Autodesk Fusion 360 part; units mm, degrees
note: some values were not read from the file. Set by a fixed rule: which sketch regions a step uses.
(part 2 of 2)
sketch "Sketch32" plane through (0, 0, 0) normal (0, -1, 0) x (1, 0, 0)
  line L0 (30, 47) -> (60, 47)
  line L1 (60, 47) -> (60, 33)
  line L2 (60, 33) -> (30, 33)
  line L3 (30, 33) -> (30, 47)
  line L4 (52, 23) -> (68, 23)
  line L5 (68, 23) -> (68, 13)
  line L6 (68, 13) -> (52, 13)
  line L7 (52, 13) -> (52, 23)
  circle A0 centre (30, 18) radius 5
  line L8 (3, 20) -> (3, 10)
  line L9 (3, 10) -> (0, 10)
  line L10 (0, 10) -> (0, 0)
  line L11 (0, 0) -> (10, 0)
  line L12 (10, 0) -> (10, 3)
  line L13 (10, 3) -> (20, 3)
  line L14 (20, 3) -> (20, 0)
  line L15 (20, 0) -> (30, 0)
  line L16 (30, 0) -> (30, 3)
  line L17 (30, 3) -> (40, 3)
  line L18 (40, 3) -> (40, 0)
  line L19 (40, 0) -> (50, 0)
  line L20 (50, 0) -> (50, 3)
  line L21 (50, 3) -> (60, 3)
  line L22 (60, 3) -> (60, 0)
  line L23 (60, 0) -> (70, 0)
  line L24 (70, 0) -> (70, 3)
  line L25 (70, 3) -> (80, 3)
  line L26 (80, 3) -> (80, 0)
  line L27 (80, 0) -> (90, 0)
  line L28 (90, 0) -> (90, 10)
  line L29 (90, 10) -> (87, 10)
  line L30 (87, 10) -> (87, 20)
  line L31 (87, 20) -> (90, 20)
  line L32 (90, 20) -> (90, 30)
  line L33 (90, 30) -> (87, 30)
  line L34 (87, 30) -> (87, 40)
  line L35 (87, 40) -> (90, 40)
  line L36 (90, 40) -> (90, 50)
  line L37 (90, 50) -> (87, 50)
  line L38 (87, 50) -> (87, 60)
  line L39 (87, 60) -> (90, 60)
  line L40 (90, 60) -> (90, 70)
  line L41 (90, 70) -> (80, 70)
  line L42 (80, 70) -> (80, 67)
  line L43 (80, 67) -> (70, 67)
  line L44 (70, 67) -> (70, 70)
  line L45 (70, 70) -> (60, 70)
  line L46 (60, 70) -> (60, 67)
  line L47 (60, 67) -> (50, 67)
  line L48 (50, 67) -> (50, 70)
  line L49 (50, 70) -> (40, 70)
  line L50 (40, 70) -> (40, 67)
  line L51 (40, 67) -> (30, 67)
  line L52 (30, 67) -> (30, 70)
  line L53 (30, 70) -> (20, 70)
  line L54 (20, 70) -> (20, 67)
  line L55 (20, 67) -> (10, 67)
  line L56 (10, 67) -> (10, 70)
  line L57 (10, 70) -> (0, 70)
  line L58 (0, 70) -> (0, 60)
  line L59 (0, 60) -> (3, 60)
  line L60 (3, 60) -> (3, 50)
  line L61 (3, 50) -> (0, 50)
  line L62 (0, 50) -> (0, 40)
  line L63 (0, 40) -> (3, 40)
  line L64 (3, 40) -> (3, 30)
  line L65 (3, 30) -> (0, 30)
  line L66 (0, 30) -> (0, 20)
  line L67 (0, 20) -> (3, 20)
  circle A1 centre (67, 43) radius 0.5
  circle A2 centre (73, 43) radius 0.5
  circle A3 centre (68.5, 43) radius 0.5
  circle A4 centre (70, 43) radius 0.5
  circle A5 centre (71.5, 43) radius 0.5
  circle A6 centre (67.75, 42) radius 0.5
  circle A7 centre (69.25, 42) radius 0.5
  circle A8 centre (70.75, 42) radius 0.5
  circle A9 centre (72.25, 42) radius 0.5
  circle A10 centre (67, 41) radius 0.5
  circle A11 centre (68.4962, 41) radius 0.5
  circle A12 centre (70, 41) radius 0.5
  circle A13 centre (71.5, 41) radius 0.5
  circle A14 centre (73, 41) radius 0.5
  circle A15 centre (67.75, 40) radius 0.5
  circle A16 centre (69.25, 40) radius 0.5
  circle A17 centre (70.75, 40) radius 0.5
  circle A18 centre (72.25, 40) radius 0.5
  circle A19 centre (67, 39) radius 0.5
  circle A20 centre (68.4962, 39) radius 0.5
  circle A21 centre (70, 39) radius 0.5
  circle A22 centre (71.5, 39) radius 0.5
  circle A23 centre (73, 39) radius 0.5
  circle A24 centre (23, 43) radius 0.5
  circle A25 centre (21.5, 43) radius 0.5
  circle A26 centre (20, 43) radius 0.5
  circle A27 centre (18.5, 43) radius 0.5
  circle A28 centre (17, 43) radius 0.5
  circle A29 centre (17.75, 42) radius 0.5
  circle A30 centre (19.25, 42) radius 0.5
  circle A31 centre (20.75, 42) radius 0.5
  circle A32 centre (22.25, 42) radius 0.5
  circle A33 centre (21.5038, 41) radius 0.5
  circle A34 centre (20, 41) radius 0.5
  circle A35 centre (18.5, 41) radius 0.5
  circle A36 centre (17, 41) radius 0.5
  circle A37 centre (17.75, 40) radius 0.5
  circle A38 centre (20.75, 40) radius 0.5
  circle A39 centre (19.25, 40) radius 0.5
  circle A40 centre (22.25, 40) radius 0.5
  circle A41 centre (23, 41) radius 0.5
  circle A42 centre (23, 39) radius 0.5
  circle A43 centre (21.5038, 39) radius 0.5
  circle A44 centre (20, 39) radius 0.5
  circle A45 centre (18.5, 39) radius 0.5
  circle A46 centre (17, 39) radius 0.5
  point P0 (70, 40)
  dimension "d174" = 1
  dimension "d175" = 1.5
  dimension "d176" = 1.5
  dimension "d177" = 1
  dimension "d178" = 1
  dimension "d179" = 1.5
  dimension "d180" = 1
  dimension "d182" = 2
  dimension "d183" = 1
  dimension "d184" = 1
  dimension "d185" = 1
  dimension "d186" = 1
  dimension "d187" = 1
  dimension "d188" = 2
  dimension "d189" = 1
  dimension "d190" = 1
  dimension "d191" = 1
  dimension "d192" = 1
  dimension "d193" = 2
  dimension "d194" = 1
  dimension "d195" = 1
  dimension "d196" = 1
  dimension "d197" = 1
  dimension "d198" = 1
  measures "d174" diameter of A6
  measures "d175" distance of A6.centre A7.centre
  measures "d176" distance of A7.centre A8.centre
  measures "d177" diameter of A7
  measures "d178" diameter of A8
  measures "d179" distance of A8.centre A9.centre
  measures "d180" diameter of A9
  measures "d182" distance of A1.centre A10.centre
  measures "d183" diameter of A10
  measures "d184" diameter of A11
  measures "d185" diameter of A12
  measures "d186" diameter of A13
  measures "d187" diameter of A14
  measures "d188" distance of A6.centre A15.centre
  measures "d189" diameter of A15
  measures "d190" diameter of A16
  measures "d191" diameter of A17
  measures "d192" diameter of A18
  measures "d193" distance of A10.centre A19.centre
  measures "d194" diameter of A19
  measures "d195" diameter of A20
  measures "d196" diameter of A21
  measures "d197" diameter of A22
  measures "d198" diameter of A23
extrude "Extrude15" cut sketch "Sketch32" against normal blind 3 contours A1 | A2 | A3 | A4 | A5 | A6 | A7 | A8 | A9 | A10 | A11 | A12 | A13 | A14 | A15 | A16 | A17 | A18 | A19 | A20 | A21 | A22 | A23 | A24 | A25 | A26 | A27 | A28 | A29 | A30 | A31 | A32 | A33 | A34 | A35 | A36 | A37 | A38 | A39 | A40 | A41 | A42 | A43 | A44 | A45 | A46 bodies 2
sketch "Sketch33" plane through (0, 3, 0) normal (0, 1, 0) x (-1, 0, 0)
  circle A0 centre (-70, 39) radius 0.5
  circle A1 centre (-70.75, 40) radius 0.5
  circle A2 centre (-68.4962, 41) radius 0.5
  circle A3 centre (-72.25, 42) radius 0.5
  circle A4 centre (-67, 43) radius 0.5
  circle A5 centre (-68.5, 43) radius 0.5
  circle A6 centre (-21.5038, 39) radius 0.5
  circle A7 centre (-20.75, 40) radius 0.5
  circle A8 centre (-20, 41) radius 0.5
  circle A9 centre (-19.25, 42) radius 0.5
  circle A10 centre (-18.5, 43) radius 0.5
  circle A11 centre (-23, 43) radius 0.5
  circle A12 centre (-17, 43) radius 0.5
  circle A13 centre (-17.75, 42) radius 0.5
  circle A14 centre (-18.5, 41) radius 0.5
  circle A15 centre (-19.25, 40) radius 0.5
  circle A16 centre (-20, 39) radius 0.5
  circle A17 centre (-70, 43) radius 0.5
  circle A18 centre (-67.75, 42) radius 0.5
  circle A19 centre (-73, 41) radius 0.5
  circle A20 centre (-67, 41) radius 0.5
  circle A21 centre (-72.25, 40) radius 0.5
  circle A22 centre (-68.4962, 39) radius 0.5
  circle A23 centre (-71.5, 39) radius 0.5
  circle A24 centre (-69.25, 40) radius 0.5
  circle A25 centre (-70, 41) radius 0.5
  circle A26 centre (-70.75, 42) radius 0.5
  circle A27 centre (-73, 43) radius 0.5
  circle A28 centre (-17, 39) radius 0.5
  circle A29 centre (-23, 39) radius 0.5
  circle A30 centre (-22.25, 40) radius 0.5
  circle A31 centre (-21.5038, 41) radius 0.5
  circle A32 centre (-20.75, 42) radius 0.5
  circle A33 centre (-20, 43) radius 0.5
  circle A34 centre (-21.5, 43) radius 0.5
  circle A35 centre (-22.25, 42) radius 0.5
  circle A36 centre (-23, 41) radius 0.5
  circle A37 centre (-17, 41) radius 0.5
  circle A38 centre (-17.75, 40) radius 0.5
  circle A39 centre (-18.5, 39) radius 0.5
  circle A40 centre (-71.5, 43) radius 0.5
  circle A41 centre (-69.25, 42) radius 0.5
  circle A42 centre (-71.5, 41) radius 0.5
  circle A43 centre (-67.75, 40) radius 0.5
  circle A44 centre (-73, 39) radius 0.5
  circle A45 centre (-67, 39) radius 0.5
  line L0 (-60, 47) -> (-30, 47)
  line L1 (-30, 47) -> (-30, 33)
  line L2 (-30, 33) -> (-60, 33)
  line L3 (-60, 33) -> (-60, 47)
  line L4 (-68, 23) -> (-52, 23)
  line L5 (-52, 23) -> (-52, 13)
  line L6 (-52, 13) -> (-68, 13)
  line L7 (-68, 13) -> (-68, 23)
  circle A46 centre (-30, 18) radius 5
  line L8 (-3, 10) -> (-3, 20)
  line L9 (-3, 20) -> (0, 20)
  line L10 (0, 20) -> (0, 30)
  line L11 (0, 30) -> (-3, 30)
  line L12 (-3, 30) -> (-3, 40)
  line L13 (-3, 40) -> (0, 40)
  line L14 (0, 40) -> (0, 50)
  line L15 (0, 50) -> (-3, 50)
  line L16 (-3, 50) -> (-3, 60)
  line L17 (-3, 60) -> (0, 60)
  line L18 (0, 60) -> (0, 70)
  line L19 (0, 70) -> (-10, 70)
  line L20 (-10, 70) -> (-10, 67)
  line L21 (-10, 67) -> (-20, 67)
  line L22 (-20, 67) -> (-20, 70)
  line L23 (-20, 70) -> (-30, 70)
  line L24 (-30, 70) -> (-30, 67)
  line L25 (-30, 67) -> (-40, 67)
  line L26 (-40, 67) -> (-40, 70)
  line L27 (-40, 70) -> (-50, 70)
  line L28 (-50, 70) -> (-50, 67)
  line L29 (-50, 67) -> (-60, 67)
  line L30 (-60, 67) -> (-60, 70)
  line L31 (-60, 70) -> (-70, 70)
  line L32 (-70, 70) -> (-70, 67)
  line L33 (-70, 67) -> (-80, 67)
  line L34 (-80, 67) -> (-80, 70)
  line L35 (-80, 70) -> (-90, 70)
  line L36 (-90, 70) -> (-90, 60)
  line L37 (-90, 60) -> (-87, 60)
  line L38 (-87, 60) -> (-87, 50)
  line L39 (-87, 50) -> (-90, 50)
  line L40 (-90, 50) -> (-90, 40)
  line L41 (-90, 40) -> (-87, 40)
  line L42 (-87, 40) -> (-87, 30)
  line L43 (-87, 30) -> (-90, 30)
  line L44 (-90, 30) -> (-90, 20)
  line L45 (-90, 20) -> (-87, 20)
  line L46 (-87, 20) -> (-87, 10)
  line L47 (-87, 10) -> (-90, 10)
  line L48 (-90, 10) -> (-90, 0)
  line L49 (-90, 0) -> (-80, 0)
  line L50 (-80, 0) -> (-80, 3)
  line L51 (-80, 3) -> (-70, 3)
  line L52 (-70, 3) -> (-70, 0)
  line L53 (-70, 0) -> (-60, 0)
  line L54 (-60, 0) -> (-60, 3)
  line L55 (-60, 3) -> (-50, 3)
  line L56 (-50, 3) -> (-50, 0)
  line L57 (-50, 0) -> (-40, 0)
  line L58 (-40, 0) -> (-40, 3)
  line L59 (-40, 3) -> (-30, 3)
  line L60 (-30, 3) -> (-30, 0)
  line L61 (-30, 0) -> (-20, 0)
  line L62 (-20, 0) -> (-20, 3)
  line L63 (-20, 3) -> (-10, 3)
  line L64 (-10, 3) -> (-10, 0)
  line L65 (-10, 0) -> (0, 0)
  line L66 (0, 0) -> (0, 10)
  line L67 (0, 10) -> (-3, 10)
sketch "Sketch34" plane through (0, 0, 0) normal (0, -1, 0) x (1, 0, 0)
  circle A0 centre (70, 39) radius 0.5
  circle A1 centre (70.75, 40) radius 0.5
  circle A2 centre (68.4962, 41) radius 0.5
  circle A3 centre (72.25, 42) radius 0.5
  circle A4 centre (67, 43) radius 0.5
  circle A5 centre (68.5, 43) radius 0.5
  circle A6 centre (21.5038, 39) radius 0.5
  circle A7 centre (20.75, 40) radius 0.5
  circle A8 centre (20, 41) radius 0.5
  circle A9 centre (19.25, 42) radius 0.5
  circle A10 centre (18.5, 43) radius 0.5
  circle A11 centre (23, 43) radius 0.5
  circle A12 centre (17, 43) radius 0.5
  circle A13 centre (17.75, 42) radius 0.5
  circle A14 centre (18.5, 41) radius 0.5
  circle A15 centre (19.25, 40) radius 0.5
  circle A16 centre (20, 39) radius 0.5
  circle A17 centre (70, 43) radius 0.5
  circle A18 centre (67.75, 42) radius 0.5
  circle A19 centre (73, 41) radius 0.5
  circle A20 centre (67, 41) radius 0.5
  circle A21 centre (72.25, 40) radius 0.5
  circle A22 centre (68.4962, 39) radius 0.5
  circle A23 centre (71.5, 39) radius 0.5
  circle A24 centre (69.25, 40) radius 0.5
  circle A25 centre (70, 41) radius 0.5
  circle A26 centre (70.75, 42) radius 0.5
  circle A27 centre (73, 43) radius 0.5
  circle A28 centre (17, 39) radius 0.5
  circle A29 centre (23, 39) radius 0.5
  circle A30 centre (22.25, 40) radius 0.5
  circle A31 centre (21.5038, 41) radius 0.5
  circle A32 centre (20.75, 42) radius 0.5
  circle A33 centre (20, 43) radius 0.5
  circle A34 centre (21.5, 43) radius 0.5
  circle A35 centre (22.25, 42) radius 0.5
  circle A36 centre (23, 41) radius 0.5
  circle A37 centre (17, 41) radius 0.5
  circle A38 centre (17.75, 40) radius 0.5
  circle A39 centre (18.5, 39) radius 0.5
  circle A40 centre (71.5, 43) radius 0.5
  circle A41 centre (69.25, 42) radius 0.5
  circle A42 centre (71.5, 41) radius 0.5
  circle A43 centre (67.75, 40) radius 0.5
  circle A44 centre (73, 39) radius 0.5
  circle A45 centre (67, 39) radius 0.5
  line L0 (30, 47) -> (60, 47)
  line L1 (60, 47) -> (60, 33)
  line L2 (60, 33) -> (30, 33)
  line L3 (30, 33) -> (30, 47)
  line L4 (52, 23) -> (68, 23)
  line L5 (68, 23) -> (68, 13)
  line L6 (68, 13) -> (52, 13)
  line L7 (52, 13) -> (52, 23)
  circle A46 centre (30, 18) radius 5
  line L8 (3, 20) -> (3, 10)
  line L9 (3, 10) -> (0, 10)
  line L10 (0, 10) -> (0, 0)
  line L11 (0, 0) -> (10, 0)
  line L12 (10, 0) -> (10, 3)
  line L13 (10, 3) -> (20, 3)
  line L14 (20, 3) -> (20, 0)
  line L15 (20, 0) -> (30, 0)
  line L16 (30, 0) -> (30, 3)
  line L17 (30, 3) -> (40, 3)
  line L18 (40, 3) -> (40, 0)
  line L19 (40, 0) -> (50, 0)
  line L20 (50, 0) -> (50, 3)
  line L21 (50, 3) -> (60, 3)
  line L22 (60, 3) -> (60, 0)
  line L23 (60, 0) -> (70, 0)
  line L24 (70, 0) -> (70, 3)
  line L25 (70, 3) -> (80, 3)
  line L26 (80, 3) -> (80, 0)
  line L27 (80, 0) -> (90, 0)
  line L28 (90, 0) -> (90, 10)
  line L29 (90, 10) -> (87, 10)
  line L30 (87, 10) -> (87, 20)
  line L31 (87, 20) -> (90, 20)
  line L32 (90, 20) -> (90, 30)
  line L33 (90, 30) -> (87, 30)
  line L34 (87, 30) -> (87, 40)
  line L35 (87, 40) -> (90, 40)
  line L36 (90, 40) -> (90, 50)
  line L37 (90, 50) -> (87, 50)
  line L38 (87, 50) -> (87, 60)
  line L39 (87, 60) -> (90, 60)
  line L40 (90, 60) -> (90, 70)
  line L41 (90, 70) -> (80, 70)
  line L42 (80, 70) -> (80, 67)
  line L43 (80, 67) -> (70, 67)
  line L44 (70, 67) -> (70, 70)
  line L45 (70, 70) -> (60, 70)
  line L46 (60, 70) -> (60, 67)
  line L47 (60, 67) -> (50, 67)
  line L48 (50, 67) -> (50, 70)
  line L49 (50, 70) -> (40, 70)
  line L50 (40, 70) -> (40, 67)
  line L51 (40, 67) -> (30, 67)
  line L52 (30, 67) -> (30, 70)
  line L53 (30, 70) -> (20, 70)
  line L54 (20, 70) -> (20, 67)
  line L55 (20, 67) -> (10, 67)
  line L56 (10, 67) -> (10, 70)
  line L57 (10, 70) -> (0, 70)
  line L58 (0, 70) -> (0, 60)
  line L59 (0, 60) -> (3, 60)
  line L60 (3, 60) -> (3, 50)
  line L61 (3, 50) -> (0, 50)
  line L62 (0, 50) -> (0, 40)
  line L63 (0, 40) -> (3, 40)
  line L64 (3, 40) -> (3, 30)
  line L65 (3, 30) -> (0, 30)
  line L66 (0, 30) -> (0, 20)
  line L67 (0, 20) -> (3, 20)
sketch "Sketch35" plane through (0, 3, 0) normal (0, 1, 0) x (-1, 0, 0)
sketch "Sketch36" plane through (0, 0, 0) normal (0, -1, 0) x (1, 0, 0)
sketch "Sketch16" plane through (0, 0, 0) normal (1, 0, 0) x (0, 1, 0)
extrude "Extrude10" [suppressed]
sketch "Sketch18" plane through (0, 0, 0) normal (0, -1, 0) x (1, 0, 0)
  line L0 (33, 25) -> (17, 25)
  line L1 (17, 25) -> (17, 15)
  line L2 (17, 15) -> (33, 15)
  line L3 (33, 15) -> (33, 25)
  line L4 (33, 25) -> (17, 15) construction
  line L5 (17, 25) -> (33, 15) construction
  point P0 (25, 20)
  constraint horizontal L0
  constraint perpendicular L0 L1
  constraint parallel L0 L2
  constraint parallel L1 L3
  constraint coincident L4 P0
  constraint coincident L5 P0
extrude "Extrude6" [suppressed]
sketch "Sketch14" plane through (0, 0, 0) normal (0, -1, 0) x (1, 0, 0)
  circle A0 centre (60, 15) radius 5
extrude "Extrude8" [suppressed]
sketch "Sketch15" plane through (0, 0, 0) normal (0, -1, 0) x (1, 0, 0)
  line L0 (20, 20) -> (36, 20)
  line L1 (36, 20) -> (36, 10)
  line L2 (36, 10) -> (20, 10)
  line L3 (20, 10) -> (20, 20)
  constraint horizontal L0
  constraint vertical L1
  constraint horizontal L2
  constraint vertical L3
extrude "Extrude9" [suppressed]
sketch "Sketch13" plane through (0, 0, 0) normal (0, -1, 0) x (1, 0, 0)
  line L0 (40, 20) -> (35, 20)
  line L1 (35, 20) -> (35, 15)
  line L2 (35, 15) -> (40, 15)
  line L3 (40, 15) -> (40, 20)
  line L4 (45, 15) -> (45, 20)
  line L5 (45, 20) -> (50, 20)
  line L6 (50, 20) -> (50, 15)
  line L7 (50, 15) -> (45, 15)
  dimension "d123" = 5
  dimension "d124" = 5
  dimension "d125" = 5
  dimension "d126" = 5
  dimension "d127" = 5
  dimension "d128" = 5
  dimension "d129" = 5
  dimension "d130" = 5
  constraint horizontal L0
  constraint perpendicular L0 L1
  constraint perpendicular L1 L2
  constraint perpendicular L0 L3
  constraint vertical L4
  constraint perpendicular L4 L5
  constraint perpendicular L5 L6
  constraint perpendicular L4 L7
  measures "d123" distance of L0.start L0.end
  measures "d124" distance of L0.end L1.end
  measures "d125" distance of L1.end L2.end
  measures "d126" distance of L2.end L0.start
  measures "d127" distance of L4.start L4.end
  measures "d128" distance of L4.end L5.end
  measures "d129" distance of L5.end L6.end
  measures "d130" distance of L6.end L4.start
extrude "Extrude7" [suppressed]
equation "Length = 90 mm"
equation "Breadth = 70 mm"
equation "Height = 70 mm"
equation "FingerL = 10 mm"
equation "d7 = Length"
equation "d8 = Height"
equation "d9 = FingerL"
equation "FingerB = 10 mm"
equation "FingerH = 10 mm"
equation "Thickness = 3 mm"
equation "d14 = Thickness"
equation "d15 = FingerL"
equation "d16 = Thickness"
equation "d17 = FingerL"
equation "d18 = Thickness"
equation "d19 = FingerL"
equation "d20 = Thickness"
equation "d21 = FingerL"
equation "d22 = Thickness"
equation "d23 = FingerL"
equation "d24 = Thickness"
equation "d25 = FingerL"
equation "d26 = Thickness"
equation "d27 = FingerL"
equation "d28 = FingerL"
equation "d29 = Thickness"
equation "d30 = FingerH"
equation "d31 = Thickness"
equation "d32 = FingerH"
equation "d33 = Thickness"
equation "d34 = FingerH"
equation "d35 = Thickness"
equation "d36 = FingerH"
equation "d37 = Thickness"
equation "d38 = FingerH"
equation "d39 = Thickness"
equation "d40 = FingerH"
equation "d41 = Thickness"
equation "d42 = FingerH"
equation "d43 = FingerL"
equation "d44 = Thickness"
equation "d45 = FingerL"
equation "d46 = Thickness"
equation "d47 = FingerL"
equation "d48 = Thickness"
equation "d49 = FingerL"
equation "d50 = Thickness"
equation "d51 = FingerL"
equation "d52 = Thickness"
equation "d53 = FingerL"
equation "d54 = Thickness"
equation "d55 = FingerL"
equation "d56 = Thickness"
equation "d57 = FingerL"
equation "d58 = Thickness"
equation "d59 = FingerL"
equation "d60 = FingerH"
equation "d61 = Thickness"
equation "d62 = FingerH"
equation "d63 = Thickness"
equation "d64 = FingerH"
equation "d65 = Thickness"
equation "d66 = FingerH"
equation "d67 = Thickness"
equation "d68 = FingerH"
equation "d69 = Thickness"
equation "d70 = FingerH"
equation "d71 = Thickness"
equation "d72 = Length"
equation "d73 = Breadth"
equation "d74 = Thickness"
equation "d76 = Thickness"
equation "d78 = -Breadth / 2"
equation "d80 = Breadth"
equation "d81 = Height"
equation "d82 = FingerB"
equation "d83 = Thickness"
equation "d84 = FingerB"
equation "d85 = Thickness"
equation "d86 = FingerB"
equation "d87 = Thickness"
equation "d88 = FingerB"
equation "d89 = Thickness"
equation "d90 = FingerB"
equation "d91 = Thickness"
equation "d93 = FingerB"
equation "d94 = Thickness"
equation "d97 = -Thickness"
equation "d99 = -Length / 2"
equation "d101 = -Height"
equation "d102 = Length"
equation "d103 = Breadth"
equation "d104 = Thickness"
equation "d120 = -Thickness / 2"
equation "Buttonsize = 5 mm"
equation "d123 = Buttonsize"
equation "d124 = Buttonsize"
equation "d125 = Buttonsize"
equation "d126 = Buttonsize"
equation "d127 = Buttonsize"
equation "d128 = Buttonsize"
equation "d129 = Buttonsize"
equation "d130 = Buttonsize"
equation "d131 = -Thickness"
equation "d133 = -Thickness"
equation "d135 = -Thickness"
equation "d138 = -Thickness"
equation "d168 = -Thickness"
equation "d199 = -Thickness"
named bodies: "Base", "Front", "Back", "Cover"
